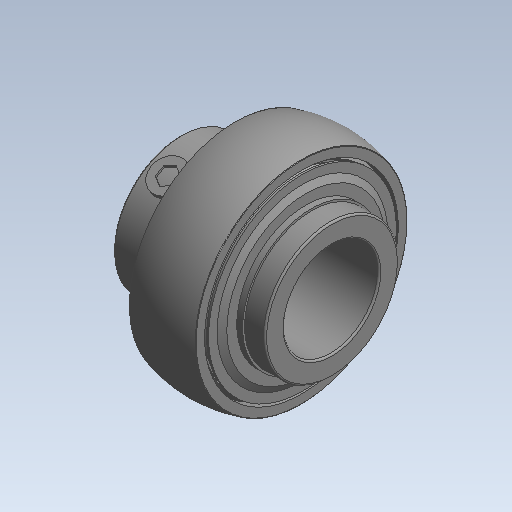
# Autodesk Inventor part: YAR 203-2F-24.210300220312 -bearing
Saved by Autodesk Inventor 2020 (Build 240168000, 168)
## iProperties
Part Number: YAR 203-2F-24.210300220312 -bearing
Material: Generic
Catalog Web Link: www.cadenas.de
Description: ayf_001hc_hh_hy_bearing-Y-bearings
Vendor: SKF
Document SubType Name: Modeling
Designer: partserver
Manufacturer: SKF
Mass: 10.89 g
Surface Area: 132.841 cm^2
Volume: 10.89 cm^3
Density: 1 g/cm^3
Appearance: PSOLRGB-175-175-175
Category: PARTsolutions
Company: SKF
PSOL_IDENT_0: {$CADENAS_DATA\23d-libs\skf\bearings_units_and_housings\bearing_units\ball_bearing_units\y-units\y-b
PSOL_IDENT_1: earing_square_flanged_units_parts\ayf_001hc_hh_hy_bearing.prj},229 {VTYP=3D},{NB=YAR 203-2F-24.21030
PSOL_IDENT_2: 0220312 -bearing},{LINA=YAR 203-2F-24.210300220312 -bearing},{NN=ayf_001hc_hh_hy_bearing},{DATE=20.0
PSOL_IDENT_3: 8.2020 13:45:20},{GEOMDATE=29.07.2020 17:09:33},{VERSION=},{LINEID=1230},{WBVAR=},{WBNUMERIC=}  {NB=
PSOL_IDENT_4: YAR 203-2F-24.210300220312 -bearing},{LINA=YAR 203-2F-24.210300220312 -bearing},{KT=DUMMY},{PRODUCTI
PSOL_IDENT_5: D=103002203},{DESIGNATION=YAR 203-2F},{DD=17.0000},{D=40},{B=27.400},{C=12.000},{PITCH=28.500},{DW=6
PSOL_IDENT_6: .747},{FO=IEC_BBY_006},{DESIGN=ybrg1},{B1=MIN},{LM=Grub screw},{DES=Inner ring extended on both side
PSOL_IDENT_7: s},{PS=For agricultural applications},{MAT=},{SS=Standard seals with additional flingers},{UNIT=Metr
PSOL_IDENT_8: ic},{G=MIN},{DD1=24.20},{DD2=MIN},{DD3=MIN},{B3=0.000},{B4=MIN},{BB4=4.0},{R12=0.3},{R12X=0},{SS1=15
PSOL_IDENT_9: .900},{NOTE=},{DG=MIN},{E=3.600},{F=1.300},{RG=MIN},{LOAD1=9.560},{LOAD2=4.750},{LOAD3=0.200},{SPEED
PSOL_IDENT_10: 2=9500},{FF0=13},{BF=1},{A15=500000},{A8=400000},{A4=300000},{BETA=1.89},{SBT1=0.094},{SBT2=},{RF1=0
PSOL_IDENT_11: .00000039},{RF2=1.7},{SF1=0.00323},{SF2=36.5},{KZ=3.1},{II=1},{Z=8},{SG=VT307},{MASS=0.10},{G2=M6x0.
PSOL_IDENT_12: 75},{HEX=3.000},{RTT=4},{MKIT=},{AS=},{TANGLE=},{SLEEVE=},{SRING=RIS 203},{FPC=RBC17_YBRG_001},{POPI=
PSOL_IDENT_13: 1},{NOUN=N020},{NOUNDES=Ball bearing},{MOD=M200},{MODDES=Radial deep groove},{YZ=12.1},{PIM=YAR 203-
PSOL_IDENT_14: 2F},{LNDD11=MIN},{LUB3=0},{BZ=0.3502},{SDALG=h},{YRZ=17.6235},{SHAPE=4},{LNB1HM11=0},{LWM=0},{TYPEID=
PSOL_IDENT_15: 103002},{LUBGR2=0},{LOCKNUT=},{LOCKDEVICE=},{LNB=MIN},{BB=MIN},{LNB1=MIN},{S1ALG=15.9},{HH=MIN},{LDB=
PSOL_IDENT_16: MIN},{LDDD1=MIN},{LDDD2=MIN},{LDM=MIN},{LDFF=MIN},{TP=4},{LNBHM11=0},{BBHM11=0},{LNDD1HM11=0},{HELP=
PSOL_IDENT_17: 5},{HHHM11=0},{LUBGR1=0},{LWV=0},{S2=21.1},{LUB2=1},{BZ1=0.000},{HEX2=}
NB: YAR 203-2F-24.210300220312 -bearing
NN: ayf_001hc_hh_hy_bearing
NT: Y-bearings
NBSYN: $DESIGNATION.-$DD1.$PRODUCTID.$C.$B1.-bearing
LINA: YAR 203-2F-24.210300220312 -bearing
CATALOG: SKF
DESIGNATION: YAR 203-2F
DD: 17
D: 40
B: 27.4
C: 12
B1: 0
DD1: 24.2
LOAD1: 9.56
LOAD2: 4.75
LOAD3: 0.2
SPEED2: 9500
SUPPLIER: SKF
ARTICLENO: YAR 203-2F-24.210300220312 -bearing
BOMINFO: YAR 203-2F-24.210300220312 -bearing
CREATOR: CADENAS GmbH
Title: YAR 203-2F-24.210300220312 -bearing
Author: Cadenas PARTsolutions
Comments: Y-bearings
Autodesk Inventor part; units mm, degrees
sketch "Sketch_1" plane through (0, 0, 0) normal (0, 0, 1) x (1, 0, 0)
  line L0 (50, 0) -> (-50, 0)
  arc A0 (-11.5, 8.8) -> (-11.2, 8.5) centre (-11.2, 8.8) ccw
  line L1 (-11.2, 8.5) -> (15.6, 8.5)
  arc A1 (15.6, 8.5) -> (15.9, 8.8) centre (15.6, 8.8) ccw
  line L2 (15.9, 8.8) -> (15.9, 11.8)
  arc A2 (15.9, 11.8) -> (15.6, 12.1) centre (15.6, 11.8) ccw
  line L3 (15.6, 12.1) -> (2.5996, 12.1)
  arc A3 (-2.5996, 12.1) -> (2.5996, 12.1) centre (0, 14.25) ccw
  line L4 (-2.5996, 12.1) -> (-11.2, 12.1)
  arc A4 (-11.2, 12.1) -> (-11.5, 11.8) centre (-11.2, 11.8) ccw
  line L5 (-11.5, 11.8) -> (-11.5, 8.8)
  constraints: 12 end point, 10 point on circle, 5 centre point
revolve "Revolution1" add sketch "Sketch_1" angle 360 about axis through (50, 0, 0) along (1, 0, 0)
sketch "Sketch_2" plane through (0, 8.5, 0) normal (0, 1, 0) x (1, 0, 0)
  circle A0 centre (11.9, 0) radius 3
  line L0 (10.4, -0.866) -> (11.9, -1.7321)
  line L1 (11.9, -1.7321) -> (13.4, -0.866)
  line L2 (13.4, -0.866) -> (13.4, 0.866)
  line L3 (13.4, 0.866) -> (11.9, 1.7321)
  line L4 (11.9, 1.7321) -> (10.4, 0.866)
  line L5 (10.4, 0.866) -> (10.4, -0.866)
  constraints: 12 end point, 1 centre point
extrude "Extrusion1" add sketch "Sketch_2" along normal blind 3.96
sketch "Sketch_3" plane through (0, -4.25, -7.3612) normal (0, -0.5, -0.8660254) x (1, 0, 0)
  circle A0 centre (11.9, 0) radius 3
  line L0 (10.4, -0.866) -> (11.9, -1.7321)
  line L1 (11.9, -1.7321) -> (13.4, -0.866)
  line L2 (13.4, -0.866) -> (13.4, 0.866)
  line L3 (13.4, 0.866) -> (11.9, 1.7321)
  line L4 (11.9, 1.7321) -> (10.4, 0.866)
  line L5 (10.4, 0.866) -> (10.4, -0.866)
  constraints: 12 end point, 1 centre point
extrude "Extrusion2" add sketch "Sketch_3" along normal blind 3.96
sketch "Sketch_4" plane through (0, 0, 0) normal (0, 0, 1) x (1, 0, 0)
  line L0 (6, 0) -> (-6, 0)
  line L1 (-7.8355, 12.4502) -> (-7.8355, 12.1)
  line L2 (-7.8355, 12.1) -> (-6.4347, 12.1)
  line L3 (-6.4347, 12.1) -> (-6.4347, 14.25)
  line L4 (-6.4347, 14.25) -> (-5.8249, 15.3745)
  line L5 (-5.8249, 15.3745) -> (-5.8249, 16.9484)
  line L6 (-5.8249, 16.9484) -> (-6.1751, 16.9484)
  line L7 (-6.1751, 16.9484) -> (-6.1751, 15.3745)
  line L8 (-6.1751, 15.3745) -> (-6.7849, 14.25)
  line L9 (-6.7849, 14.25) -> (-6.7849, 12.4502)
  line L10 (-6.7849, 12.4502) -> (-7.8355, 12.4502)
  constraints: 22 end point
revolve "Revolution2" add sketch "Sketch_4" angle 360 about axis through (6, 0, 0) along (1, 0, 0)
sketch "Sketch_5" plane through (0, 0, 0) normal (0, 0, 1) x (1, 0, 0)
  line L0 (6, 0) -> (-6, 0)
  line L1 (5.8249, 16.9484) -> (5.8249, 15.3745)
  line L2 (5.8249, 15.3745) -> (6.4347, 14.25)
  line L3 (6.4347, 14.25) -> (6.4347, 12.1)
  line L4 (6.4347, 12.1) -> (7.8355, 12.1)
  line L5 (7.8355, 12.1) -> (7.8355, 12.4502)
  line L6 (7.8355, 12.4502) -> (6.7849, 12.4502)
  line L7 (6.7849, 12.4502) -> (6.7849, 14.25)
  line L8 (6.7849, 14.25) -> (6.1751, 15.3745)
  line L9 (6.1751, 15.3745) -> (6.1751, 16.9484)
  line L10 (6.1751, 16.9484) -> (5.8249, 16.9484)
  constraints: 22 end point
revolve "Revolution3" add sketch "Sketch_5" angle 360 about axis through (6, 0, 0) along (1, 0, 0)
sketch "Sketch_6" plane through (0, 0, 0) normal (0, 0, 1) x (1, 0, 0)
  line L0 (50, 0) -> (-50, 0)
  line L1 (-6, 14.8219) -> (-6, 12.4314)
  line L2 (-6, 12.4314) -> (-5.6498, 12.4314)
  line L3 (-5.6498, 12.4314) -> (-5.6498, 14.6381)
  line L4 (-5.6498, 14.6381) -> (-4.1942, 15.643)
  line L5 (-4.1942, 15.643) -> (-4.1544, 15.5854)
  line L6 (-4.1544, 15.5854) -> (-5.5798, 14.6014)
  line L7 (-5.5798, 14.6014) -> (-5.5798, 12.5971)
  line L8 (-5.5798, 12.5971) -> (-4.2607, 12.5971)
  line L9 (-4.2607, 12.5971) -> (-4.3657, 12.1)
  line L10 (-4.3657, 12.1) -> (-4.0155, 12.1)
  line L11 (-4.0155, 12.1) -> (-3.8988, 12.6524)
  line L12 (-3.8988, 12.6524) -> (-3.8988, 13.2047)
  line L13 (-3.8988, 13.2047) -> (-4.3657, 13.757)
  line L14 (-4.3657, 13.757) -> (-4.3657, 14.8618)
  line L15 (-4.3657, 14.8618) -> (-3.8988, 15.4141)
  line L16 (-3.8988, 15.4141) -> (-3.8988, 17.5068)
  arc A0 (-3.8988, 17.5068) -> (-4.0155, 17.6235) centre (-4.0155, 17.5068) ccw
  line L17 (-4.0155, 17.6235) -> (-4.1323, 17.6235)
  arc A1 (-4.1323, 17.6235) -> (-4.249, 17.5068) centre (-4.1323, 17.5068) ccw
  line L18 (-4.249, 17.5068) -> (-4.8675, 16.7697)
  line L19 (-4.8675, 16.7697) -> (-4.5992, 16.5446)
  line L20 (-4.5992, 16.5446) -> (-4.249, 16.962)
  line L21 (-4.249, 16.962) -> (-4.249, 16.0307)
  line L22 (-4.249, 16.0307) -> (-6, 14.8219)
  constraints: 46 end point, 4 point on circle, 2 centre point
revolve "Revolution4" add sketch "Sketch_6" angle 360 about axis through (50, 0, 0) along (1, 0, 0)
sketch "Sketch_11" plane through (0, 0, 0) normal (0, 0, 1) x (1, 0, 0)
  line L0 (50, 0) -> (-50, 0)
  line L1 (3.8988, 17.5068) -> (3.8988, 15.4141)
  line L2 (3.8988, 15.4141) -> (4.3657, 14.8618)
  line L3 (4.3657, 14.8618) -> (4.3657, 13.757)
  line L4 (4.3657, 13.757) -> (3.8988, 13.2047)
  line L5 (3.8988, 13.2047) -> (3.8988, 12.6524)
  line L6 (3.8988, 12.6524) -> (4.0155, 12.1)
  line L7 (4.0155, 12.1) -> (4.3657, 12.1)
  line L8 (4.3657, 12.1) -> (4.2607, 12.5971)
  line L9 (4.2607, 12.5971) -> (5.5798, 12.5971)
  line L10 (5.5798, 12.5971) -> (5.5798, 14.6014)
  line L11 (5.5798, 14.6014) -> (4.1544, 15.5854)
  line L12 (4.1544, 15.5854) -> (4.1942, 15.643)
  line L13 (4.1942, 15.643) -> (5.6498, 14.6381)
  line L14 (5.6498, 14.6381) -> (5.6498, 12.4314)
  line L15 (5.6498, 12.4314) -> (6, 12.4314)
  line L16 (6, 12.4314) -> (6, 14.8219)
  line L17 (6, 14.8219) -> (4.249, 16.0307)
  line L18 (4.249, 16.0307) -> (4.249, 16.962)
  line L19 (4.249, 16.962) -> (4.5992, 16.5446)
  line L20 (4.5992, 16.5446) -> (4.8675, 16.7697)
  line L21 (4.8675, 16.7697) -> (4.249, 17.5068)
  arc A0 (4.249, 17.5068) -> (4.1323, 17.6235) centre (4.1323, 17.5068) ccw
  line L22 (4.1323, 17.6235) -> (4.0155, 17.6235)
  arc A1 (4.0155, 17.6235) -> (3.8988, 17.5068) centre (4.0155, 17.5068) ccw
  constraints: 46 end point, 4 point on circle, 2 centre point
revolve "Revolution5" add sketch "Sketch_11" angle 360 about axis through (50, 0, 0) along (1, 0, 0)
sketch "Sketch_16" plane through (0, 0, 0) normal (0, 0, 1) x (1, 0, 0)
  line L0 (6, 0) -> (-6, 0)
  line L1 (-6, 17.4734) -> (-4.3224, 17.4734)
  line L2 (-4.3224, 17.4734) -> (-4.1889, 17.5748)
  arc A0 (-3.8872, 17.4594) -> (-4.1889, 17.5748) centre (-4.0739, 17.4234) ccw
  line L3 (-3.8872, 17.4594) -> (-3.82, 17.1109)
  arc A1 (-3.82, 17.1109) -> (-3.6236, 16.9488) centre (-3.6236, 17.1488) ccw
  line L4 (-3.6236, 16.9488) -> (-2.1071, 16.9488)
  arc A2 (-2.1071, 16.9488) -> (-1.9595, 16.996) centre (-2.1071, 17.2028) ccw
  arc A3 (1.9595, 16.996) -> (-1.9595, 16.996) centre (0, 14.25) ccw
  arc A4 (1.9595, 16.996) -> (2.1071, 16.9488) centre (2.1071, 17.2028) ccw
  line L5 (2.1071, 16.9488) -> (3.6236, 16.9488)
  arc A5 (3.6236, 16.9488) -> (3.82, 17.1109) centre (3.6236, 17.1488) ccw
  line L6 (3.82, 17.1109) -> (3.8872, 17.4594)
  arc A6 (4.1889, 17.5748) -> (3.8872, 17.4594) centre (4.0739, 17.4234) ccw
  line L7 (4.1889, 17.5748) -> (4.3224, 17.4734)
  line L8 (4.3224, 17.4734) -> (6, 17.4734)
  line L9 (6, 17.4734) -> (6, 19.0053)
  arc A7 (6, 19.0053) -> (5.9296, 19.1008) centre (5.9, 19.0053) ccw
  arc A8 (5.9296, 19.1008) -> (-5.9296, 19.1008) centre (0, 0) ccw
  arc A9 (-5.9296, 19.1008) -> (-6, 19.0053) centre (-5.9, 19.0053) ccw
  line L10 (-6, 19.0053) -> (-6, 17.4734)
  constraints: 22 end point, 20 point on circle, 10 centre point
revolve "Revolution6" add sketch "Sketch_16" angle 360 about axis through (6, 0, 0) along (1, 0, 0)
sketch "Sketch_21" plane through (0, 0, 0) normal (0, 0, 1) x (1, 0, 0)
  line L0 (-2.9253, 14.25) -> (-2.9253, 28.5)
  line L1 (-2.9253, 28.5) -> (-2.2753, 28.5)
  line L2 (-2.2753, 28.5) -> (-2.2753, 14.25)
  line L3 (-2.2753, 14.25) -> (-2.9253, 14.25)
  line L4 (-2.9253, 14.25) -> (-2.9253, 28.5)
  constraints: 10 end point
revolve "Revolution7" cut sketch "Sketch_21" angle 360 about axis through (-2.9253, 14.25, 0) along (0, -1, 0)
ref_plane "ball_1_XY" through (0, 14.25, 0) normal (1, 0, 0) x (0, 0, -1)
ref_plane "ball_1_YZ" through (0, 14.25, 0) normal (0, 0, -1) x (0, 1, 0)
ref_plane "ball_1_ZX" through (0, 14.25, 0) normal (0, 1, 0) x (1, 0, 0)
ref_plane "ball_2_XY" through (0, 10.0763, 10.0763) normal (1, 0, 0) x (0, 0, -1)
ref_plane "ball_2_YZ" through (0, 10.0763, 10.0763) normal (0, 0, -1) x (0, 1, 0)
ref_plane "ball_2_ZX" through (0, 10.0763, 10.0763) normal (0, 1, 0) x (1, 0, 0)
ref_plane "ball_3_XY" through (0, 0, 14.25) normal (1, 0, 0) x (0, 0, -1)
ref_plane "ball_3_YZ" through (0, 0, 14.25) normal (0, 0, -1) x (0, 1, 0)
ref_plane "ball_3_ZX" through (0, 0, 14.25) normal (0, 1, 0) x (1, 0, 0)
ref_plane "ball_4_XY" through (0, -10.0763, 10.0763) normal (1, 0, 0) x (0, 0, -1)
ref_plane "ball_4_YZ" through (0, -10.0763, 10.0763) normal (0, 0, -1) x (0, 1, 0)
ref_plane "ball_4_ZX" through (0, -10.0763, 10.0763) normal (0, 1, 0) x (1, 0, 0)
ref_plane "ball_5_XY" through (0, -14.25, 0) normal (1, 0, 0) x (0, 0, -1)
ref_plane "ball_5_YZ" through (0, -14.25, 0) normal (0, 0, -1) x (0, 1, 0)
ref_plane "ball_5_ZX" through (0, -14.25, 0) normal (0, 1, 0) x (1, 0, 0)
ref_plane "ball_6_XY" through (0, -10.0763, -10.0763) normal (1, 0, 0) x (0, 0, -1)
ref_plane "ball_6_YZ" through (0, -10.0763, -10.0763) normal (0, 0, -1) x (0, 1, 0)
ref_plane "ball_6_ZX" through (0, -10.0763, -10.0763) normal (0, 1, 0) x (1, 0, 0)
ref_plane "ball_7_XY" through (0, 0, -14.25) normal (1, 0, 0) x (0, 0, -1)
ref_plane "ball_7_YZ" through (0, 0, -14.25) normal (0, 0, -1) x (0, 1, 0)
ref_plane "ball_7_ZX" through (0, 0, -14.25) normal (0, 1, 0) x (1, 0, 0)
ref_plane "ball_8_XY" through (0, 10.0763, -10.0763) normal (1, 0, 0) x (0, 0, -1)
ref_plane "ball_8_YZ" through (0, 10.0763, -10.0763) normal (0, 0, -1) x (0, 1, 0)
ref_plane "ball_8_ZX" through (0, 10.0763, -10.0763) normal (0, 1, 0) x (1, 0, 0)
ref_plane "brg_XY" through (0, 0, 0) normal (1, 0, 0) x (0, 0, -1)
ref_plane "brg_YZ" through (0, 0, 0) normal (0, 0, -1) x (0, 1, 0)
ref_plane "brg_ZX" through (0, 0, 0) normal (0, 1, 0) x (1, 0, 0)
ref_plane "brg3_XY" through (15.9, 0, 0) normal (1, 0, 0) x (0, 0, -1)
ref_plane "brg3_YZ" through (15.9, 0, 0) normal (0, 0, -1) x (0, 1, 0)
ref_plane "brg3_ZX" through (15.9, 0, 0) normal (0, 1, 0) x (1, 0, 0)
body "Solid1"
